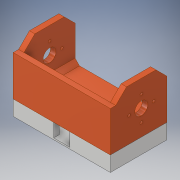
# Autodesk Inventor part: Platform
Saved by Autodesk Inventor 2019.2 (Build 232265000, 265)
## iProperties
Created: 2019-05-20
Part Number: Platform
Material: Generic
Document SubType Name: Modeling
Designer: Johansson
Density: 1 g/cm^3
Appearance: Default
Author: Johansson
Autodesk Inventor part; units mm, degrees
ref_plane "YZ Plane" through (0, 0, 0) normal (1, 0, 0) x (0, 1, 0)
ref_plane "XZ Plane" through (0, 0, 0) normal (0, 1, 0) x (-1, 0, 0)
ref_plane "XY Plane" through (0, 0, 0) normal (0, 0, 1) x (1, 0, 0)
sketch "Sketch1" plane through (0, 0, 0) normal (0, 1, 0) x (-1, 0, 0)
  line L0 (80, 47.25) -> (-80, 47.25)
  line L1 (-80, 47.25) -> (-80, -47.25)
  line L2 (-80, -47.25) -> (80, -47.25)
  line L3 (80, -47.25) -> (80, 47.25)
  line L4 (80, 47.25) -> (-80, -47.25) construction
  line L5 (-80, 47.25) -> (80, -47.25) construction
  point P0 (0, 0)
  dimension "d0" = 160
  dimension "d1" = 94.5
  constraints: 12 end point, 2 midpoint, 2 parallel, 1 horizontal, 1 perpendicular
  measures "d0" distance of L1.end L2.end
  measures "d1" distance between parallel lines of L0 L2
extrude "Extrusion1" add sketch "Sketch1" along normal blind 10
sketch "Sketch2" plane through (-80, 0, -47.25) normal (-1, 0, 0) x (0, 0, 1)
  line L0 (94.5, 0) -> (0, 0)
  line L1 (0, 0) -> (0, 94.5)
  line L2 (0, 94.5) -> (94.5, 94.5)
  line L3 (94.5, 94.5) -> (94.5, 0)
  line L4 (94.5, 0) -> (0, 94.5) construction
  line L5 (0, 0) -> (94.5, 94.5) construction
  line L6 (0, 0) -> (0, 10) projected
  line L7 (94.5, 0) -> (94.5, 10) projected
  line L8 (0, 0) -> (94.5, 0) projected
  line L9 (47.25, -15.12) -> (47.25, 90.72) projected
  line L10 (0, 10) -> (94.5, 10) projected
  circle A0 centre (47.25, 69.25) radius 2.5
  circle A1 centre (24.5, 46.5) radius 2.5
  circle A2 centre (47.25, 23.75) radius 2.5
  circle A3 centre (70, 46.5) radius 2.5
  circle A4 centre (47.25, 46.5) radius 12
  point P0 (47.25, 0)
  point P1 (47.25, 47.25)
  dimension "d4" = 94.5
  dimension "d7" = 36.5
  dimension "d10" = 360
  dimension "d12" = 5
  dimension "d13" = 22.75
  dimension "d14" = 24
  constraints: 12 end point, 5 centre point, 3 collinear, 2 midpoint, 2 parallel, 2 point on line, 1 coincident, 1 horizontal, 1 perpendicular, 9 other
  measures "d4" distance between parallel lines of L2 L0
  measures "d7" distance from line of L10 point (47.25, 46.5)
  measures "d12" diameter of A0
  measures "d13" distance of A0.centre point (47.25, 46.5)
  measures "d14" diameter of A4
extrude "Extrusion2" add sketch "Sketch2" along normal blind 10
mirror "Mirror2" about plane through (0, 0, 0) normal (1, 0, 0) of "Extrusion2"
chamfer "Chamfer1" distance 20 angle 45 4 edges at (85, 94.5, 47.25) (85, 94.5, -47.25) (-85, 94.5, 47.25) (-85, 94.5, -47.25)
chamfer "Chamfer2" distance 8.25 angle 45 2 edges at (80, 10, 0) (-80, 10, 0)
sketch "Sketch4" plane through (-90, 0, 47.25) normal (0, 0, 1) x (1, 0, 0)
  line L0 (0, 74.5) -> (180, 74.5)
  line L1 (180, 74.5) -> (180, 0)
  line L2 (180, 0) -> (0, 0)
  line L3 (0, 0) -> (0, 74.5)
  line L4 (0, 74.5) -> (180, 0) construction
  line L5 (180, 74.5) -> (0, 0) construction
  line L6 (180, 0) -> (180, 74.5) projected
  line L7 (0, 0) -> (0, 74.5) projected
  line L8 (0, 0) -> (180, 0) projected
  line L9 (0, 74.5) -> (10, 74.5) projected
  point P0 (90, 0)
  point P1 (90, 37.25)
  constraints: 12 end point, 4 collinear, 2 midpoint, 2 parallel, 1 horizontal, 1 perpendicular
extrude "Extrusion3" add sketch "Sketch4" along normal blind 10
sketch "Sketch5" plane through (0, 0, 0) normal (0, -1, 0) x (1, 0, 0)
  line L0 (90, -47.25) -> (80, -47.25)
  line L1 (80, -47.25) -> (80, 47.25)
  line L2 (80, 47.25) -> (15, 47.25)
  line L3 (15, 47.25) -> (15, 57.25)
  line L4 (15, 57.25) -> (90, 57.25)
  line L5 (90, 57.25) -> (90, -47.25)
  line L6 (0, -68.15) -> (0, 78.15) projected
  line L7 (-90, -47.25) -> (-80, -47.25)
  line L8 (-80, -47.25) -> (-80, 47.25)
  line L9 (-80, 47.25) -> (-15, 47.25)
  line L10 (-15, 47.25) -> (-15, 57.25)
  line L11 (-15, 57.25) -> (-90, 57.25)
  line L12 (-90, 57.25) -> (-90, -47.25)
  line L13 (-90, -47.25) -> (-90, 57.25) projected
  line L14 (-90, 57.25) -> (90, 57.25) projected
  line L15 (-90, -47.25) -> (90, -47.25) projected
  point P0 (0, 0)
  dimension "d23" = 10
  dimension "d24" = 10
  dimension "d25" = 30
  constraints: 24 end point, 6 symmetric about line, 5 perpendicular, 3 collinear, 1 horizontal
  measures "d23" distance of L0.start L0.end
  measures "d24" distance between parallel lines of L2 L4
  measures "d25" distance between parallel lines of L10 L3
extrude "Extrusion4" add sketch "Sketch5" along normal blind 25 separate body contours L0 L1 L2 L3 L4 L5 | L7 L12 L11 L10 L9 L8
sketch "Sketch6" plane through (0, -25, 0) normal (0, -1, 0) x (1, 0, 0)
  line L0 (-15, 57.25) -> (-90, 57.25) projected
  line L1 (90, -47.25) -> (-90, -47.25)
  line L2 (-90, -47.25) -> (-90, 57.25)
  line L3 (-90, 57.25) -> (90, 57.25)
  line L4 (90, 57.25) -> (90, -47.25)
  line L5 (90, -47.25) -> (-90, 57.25) construction
  line L6 (-90, -47.25) -> (90, 57.25) construction
  line L7 (90, -47.25) -> (90, 57.25) projected
  line L8 (80, -47.25) -> (90, -47.25) projected
  point P0 (0, 0)
  point P1 (0, 5)
  constraints: 12 end point, 2 collinear, 2 midpoint, 2 parallel, 1 horizontal, 1 perpendicular
extrude "Extrusion5" add sketch "Sketch6" along normal blind 3 bodies 2
equation "\"d0\" = 2.5 * WO_BLDC"
equation "\"d1\" = 1.5 * DO_BLDC"
equation "\"d4\" = 1.5 * DO_BLDC"
equation "\"d13\" = 0.5 * D_Hole_BLDC"
equation "\"d14\" = 3 * D_Shaft_BLDC"
equation "\"d24\" = d23"
equation "\"DO_BLDC\" = 63"
equation "\"WO_BLDC\" = 64"
equation "\"D_Shaft_BLDC\" = 8"
equation "\"D_Hole_BLDC\" = 45.5"
equation "\"D_Wheel\" = 235"
body "Solid1"
body "Solid2"
